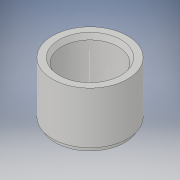
# Autodesk Inventor part: Lozysko GSM-0608-06
Saved by Autodesk Inventor 2019 (Build 230136000, 136)
## iProperties
Created: 2022-09-22
Part Number: Lozysko GSM-0608-06
Material: Ogólny
Document SubType Name: Modeling
Designer: Michał
Density: 1 g/cm^3
Appearance: Domyślna
Author: Michał
Autodesk Inventor part; units mm, degrees
ref_plane "YZ Plane" through (0, 0, 0) normal (1, 0, 0) x (0, 1, 0)
ref_plane "XZ Plane" through (0, 0, 0) normal (0, 1, 0) x (-1, 0, 0)
ref_plane "XY Plane" through (0, 0, 0) normal (0, 0, 1) x (1, 0, 0)
sketch "Szkic1" plane through (0, 0, 0) normal (0, 0, 1) x (1, 0, 0)
  line L0 (0, 0) -> (3, 0) construction
  line L1 (3, 0) -> (3, 5.5)
  line L2 (3, 5.5) -> (3.2887, 6)
  line L3 (3.2887, 6) -> (4, 6)
  line L4 (4, 6) -> (4, 0.5)
  line L5 (4, 0.5) -> (3.7113, 0)
  line L6 (3.7113, 0) -> (3, 0)
  line L7 (0, -1.2) -> (0, 7.2) projected
  dimension "d0" = 3
  dimension "d1" = 4
  dimension "d2" = 30
  dimension "d4" = 6
  dimension "d5" = 0.5
  constraints: 14 end point, 3 parallel, 2 horizontal, 1 perpendicular, 1 vertical
  measures "d0" distance of L0.end L0.start
  measures "d1" distance from line of L4 L0.start
  measures "d2" angle of L4 L5
  measures "d4" distance from line of L3.end L0
  measures "d5" distance from line of L0 L4.end
revolve "Obrót1" add sketch "Szkic1" angle 360 about axis through (0, -10, 0) along (0, 1, 0)
